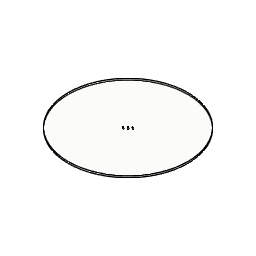
turn-table v2 (Autodesk Fusion 360 design; units mm, degrees)
Autodesk Fusion 360 part; units mm, degrees
sketch "Sketch1" plane through (0, 0, 0) normal (0, 0, 1) x (1, 0, 0)
  circle A0 centre (0, 0) radius 190.5
  circle A1 centre (0, 0) radius 2.5
  line L0 (0, 0) -> (9.5776, 8.3403)
  line L1 (9.5776, 8.3403) -> (8.0693, 7.0268)
  circle A2 centre (8.0693, 7.0268) radius 2
  line L2 (0, 0) -> (-9.5776, -8.3403)
  line L3 (-9.5776, -8.3403) -> (-8.0693, -7.0268)
  circle A3 centre (-8.0693, -7.0268) radius 2
  dimension "d1" = 381
  dimension "d2" = 5
  dimension "d3" = 12.7
  dimension "d4" = 2
  dimension "d5" = 12.7
  dimension "d6" = 2
  dimension "d7" = 4
  constraint coincident A0.centre A1.centre
  constraint concentric A0 A1
  constraint coincident L0 L1.end
  constraint coincident L1.end A2.centre
  constraint coincident L0.end A2
  constraint parallel L0 L2
  constraint parallel L2 L3
  constraint coincident L3.end A3.centre
  measures "d1" diameter of A0
  measures "d2" diameter of A1
  measures "d3" distance of A0.centre L0.end
  measures "d4" distance of L0.end L1.end
  measures "d5" distance of A0.centre L2.end
  measures "d6" distance of L2.end L3.end
  measures "d7" diameter of A3
extrude "Extrude1" add sketch "Sketch1" along normal blind 5
